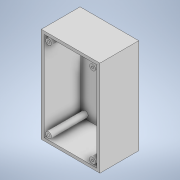
# Autodesk Inventor part: theMonarchPCBHolder
Saved by Autodesk Inventor 2020 (Build 240168000, 168)
## iProperties
Created: 2020-10-14
Part Number: theMonarchPCBHolder
Material: Generic
Document SubType Name: Modeling
Designer: s4393944
Density: 1 g/cm^3
Appearance: Default
Author: s4393944
Autodesk Inventor part; units mm, degrees
ref_plane "YZ Plane" through (0, 0, 0) normal (1, 0, 0) x (0, 1, 0)
ref_plane "XZ Plane" through (0, 0, 0) normal (0, 1, 0) x (-1, 0, 0)
ref_plane "XY Plane" through (0, 0, 0) normal (0, 0, 1) x (1, 0, 0)
sketch "Sketch1" plane through (0, 0, 0) normal (0, 0, 1) x (1, 0, 0)
  line L0 (40, -65) -> (-40, -65)
  line L1 (-40, -65) -> (-40, 65)
  line L2 (-40, 65) -> (40, 65)
  line L3 (40, 65) -> (40, -65)
  line L4 (40, -65) -> (-40, 65) construction
  line L5 (-40, -65) -> (40, 65) construction
  point P0 (0, 0)
  dimension "d0" = 80
  dimension "d1" = 130
  constraints: 12 end point, 2 midpoint, 2 parallel, 1 horizontal, 1 perpendicular
  measures "d0" distance of L1.end L2.end
  measures "d1" distance of L0.end L1.end
extrude "Extrusion1" add sketch "Sketch1" along normal blind 3
sketch "Sketch4" plane through (0, 0, 3) normal (0, 0, 1) x (1, 0, 0)
  line L0 (26.4795, -48.7045) -> (-26.4795, 48.7045) construction
  line L1 (-26.4795, -48.7045) -> (26.4795, 48.7045) construction
  circle A0 centre (-22.7965, 45.2755) radius 1.5
  circle A1 centre (23.0505, -45.2755) radius 1.5
  circle A2 centre (-22.7965, 45.2755) radius 4
  circle A3 centre (23.0505, -45.2755) radius 4
  point P0 (0, 0)
  dimension "d13" = 52.959
  dimension "d14" = 97.409
  dimension "d17" = 3
  dimension "d20" = 3
  dimension "d36" = 8
  dimension "d37" = 8
  constraints: 4 centre point, 4 end point, 2 coincident, 2 midpoint
  measures "d13" distance of L0.end L1.end
  measures "d14" distance of L1.start L0.end
  measures "d17" diameter of A0
  measures "d20" diameter of A1
  measures "d36" diameter of A2
  measures "d37" diameter of A3
sketch "Sketch5" plane through (0, 0, 3) normal (0, 0, 1) x (1, 0, 0)
  line L0 (-40, 65) -> (-40, -65) projected
  line L1 (40, -65) -> (-40, -65)
  line L2 (-40, -65) -> (-40, 65)
  line L3 (40, 65) -> (40, -65)
  line L4 (36, -61) -> (-36, -61)
  line L5 (-36, -61) -> (-36, 61)
  line L6 (-36, 61) -> (36, 61)
  line L7 (36, 61) -> (36, -61)
  line L8 (40, 65) -> (-40, 65) projected
  line L9 (40, 65) -> (-40, 65)
  line L10 (-40, -65) -> (40, -65) projected
  point P0 (0, 0)
  dimension "d28" = 72
  dimension "d29" = 122
  dimension "d30" = 61
  dimension "d33" = 36
  dimension "d34" = 130
  dimension "d35" = 80
  dimension "d50" = 0
  constraints: 16 end point, 3 parallel, 2 horizontal, 2 perpendicular
  measures "d28" distance of L5.end L6.end
  measures "d29" distance of L6.end L4.start
  measures "d30" distance from line of L6 point (0, 0)
  measures "d33" distance from line of L7 point (0, 0)
  measures "d34" distance of L3.start L1.start
  measures "d35" distance of L1.start L1.end
  measures "d50" distance between parallel lines of L10 L1
extrude "Extrusion4" add sketch "Sketch5" along normal blind 50
extrude "Extrusion5" add sketch "Sketch4" along normal blind 8
sketch "Sketch7" plane through (-22.7965, 45.2755, 11) normal (0, 0, 1) x (1, 0, 0)
  circle A0 centre (0, 0) radius 2.8
  point P0 (22.7965, -45.2755)
  dimension "d40" = 5.6
  constraints: 1 centre point
  measures "d40" diameter of A0
extrude "Extrusion6" cut sketch "Sketch7" against normal blind 3
sketch "Sketch8" plane through (23.0505, -45.2755, 11) normal (0, 0, 1) x (1, 0, 0)
  circle A0 centre (0, 0) radius 2.8
  point P0 (-23.0505, 45.2755)
  dimension "d43" = 5.6
  constraints: 1 centre point
  measures "d43" diameter of A0
extrude "Extrusion7" cut sketch "Sketch8" against normal blind 3
sketch "Sketch11" plane through (0, 0, 3) normal (0, 0, 1) x (1, 0, 0)
  circle A0 centre (-30, 55) radius 4
  circle A1 centre (30, 55) radius 4
  circle A2 centre (30, -55) radius 4
  circle A3 centre (-30, -55) radius 4
  line L0 (40, 65) -> (-40, 65) projected
  line L1 (-40, -65) -> (40, -65) projected
  circle A4 centre (-30, 55) radius 1.5
  circle A5 centre (30, 55) radius 1.5
  circle A6 centre (-30, -55) radius 1.5
  circle A7 centre (30, -55) radius 1.5
  point P0 (0, 0)
  dimension "d51" = 8
  dimension "d52" = 8
  dimension "d53" = 8
  dimension "d54" = 8
  dimension "d55" = 10
  dimension "d56" = 10
  dimension "d57" = 10
  dimension "d58" = 10
  dimension "d59" = 30
  dimension "d60" = 30
  dimension "d61" = 30
  dimension "d62" = 30
  dimension "d63" = 3
  dimension "d64" = 3
  dimension "d65" = 3
  dimension "d66" = 3
  constraints: 8 centre point, 4 coincident
  measures "d51" diameter of A0
  measures "d52" diameter of A1
  measures "d53" diameter of A2
  measures "d54" diameter of A3
  measures "d55" distance from line of L0 A0.centre
  measures "d56" distance from line of L0 A1.centre
  measures "d57" distance from line of L1 A3.centre
  measures "d58" distance from line of L1 A2.centre
  measures "d59" horizontal distance of point (0, 0) A0.centre
  measures "d60" horizontal distance of A1.centre point (0, 0)
  measures "d61" horizontal distance of point (0, 0) A2.centre
  measures "d62" horizontal distance of A3.centre point (0, 0)
  measures "d63" diameter of A4
  measures "d64" diameter of A5
  measures "d65" diameter of A6
  measures "d66" diameter of A7
extrude "Extrusion8" add sketch "Sketch11" along normal blind 50
body "Solid1"
